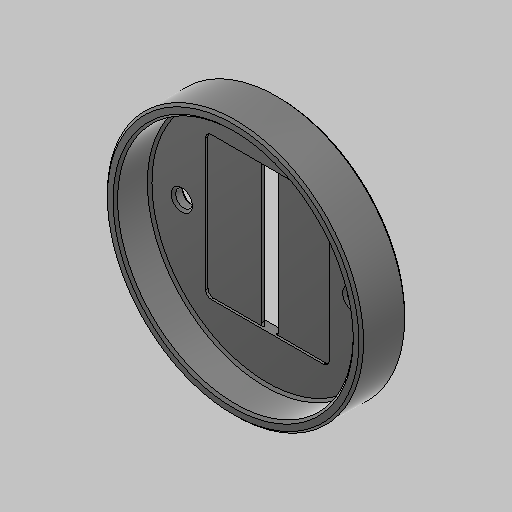
# Autodesk Inventor part: takumar-slit
Saved by Autodesk Inventor 2026 (Build 300175050, 175E)
## iProperties
Created: 2025-11-07
Part Number: takumar-slit
Material: ABS Plastic
Document SubType Name: Modeling
Designer: queezz
Density: 1.06 g/cm^3
Appearance: Smooth - Black
Author: queezz
Autodesk Inventor part; units mm, degrees
ref_plane "YZ Plane" through (0, 0, 0) normal (1, 0, 0) x (0, 1, 0)
ref_plane "XZ Plane" through (0, 0, 0) normal (0, 1, 0) x (-1, 0, 0)
ref_plane "XY Plane" through (0, 0, 0) normal (0, 0, 1) x (1, 0, 0)
sketch "Sketch1" plane through (0, 0, 0) normal (0, 0, 1) x (1, 0, 0)
  circle A0 centre (0, 0) radius 20.6
  circle A1 centre (0, 0) radius 22.4
  dimension "d0" = 41.2
  dimension "d1" = 1.8
  constraints: 2 centre point, 2 coincident
  measures "d0" diameter of A0
  measures "d1" radial gap between concentric circles of A0 A1
extrude "Extrusion1" add sketch "Sketch1" along normal blind 2 contours A0 | A1
extrude "Extrusion2" add sketch "Sketch1" along normal blind 8
sketch "Sketch2" plane through (0, 0, 2) normal (0, 0, 1) x (1, 0, 0)
  line L0 (-1.5, 12.5) -> (1.5, 12.5)
  line L1 (1.5, 12.5) -> (1.5, -12.5)
  line L2 (1.5, -12.5) -> (-1.5, -12.5)
  line L3 (-1.5, -12.5) -> (-1.5, 12.5)
  point P0 (0, 0)
  point P1 (0, 12.5)
  point P2 (1.5, 0)
  dimension "d6" = 3
  dimension "d7" = 25
  constraints: 8 end point, 2 midpoint, 2 parallel, 1 horizontal, 1 horizontal alignment, 1 perpendicular, 1 vertical alignment
  measures "d6" distance of L0.start L0.end
  measures "d7" distance of L0.end L1.end
extrude "Extrusion3" cut sketch "Sketch2" against normal through all
sketch "Sketch3" plane through (0, 0, 2) normal (0, 0, 1) x (1, 0, 0)
  line L0 (1.5, 12.5) -> (1.5, -12.5) projected
  line L1 (1.5, 12.5) -> (10.8, 12.5)
  line L2 (10.8, 12.5) -> (10.8, -12.5)
  line L3 (10.8, -12.5) -> (1.5, -12.5)
  line L4 (1.5, -12.5) -> (1.5, 12.5)
  point P0 (0, 0)
  dimension "d10" = 9.3
  constraints: 8 end point, 2 parallel, 1 horizontal, 1 perpendicular
  measures "d10" distance of L0.start L1.end
extrude "Extrusion4" cut sketch "Sketch3" against normal blind 0.4
mirror "Mirror1" about plane through (0, 0, 0) normal (1, 0, 0) of "Extrusion4"
chamfer "Chamfer1" distance 1 angle 45 2 edges at (1.5, 0, 0) (-1.5, 0, 0)
fillet "Fillet1" radius 0.4 4 edges at (-1.5, -12.5, 1.3) (1.5, -12.5, 1.3) (-1.5, 12.5, 1.3) (1.5, 12.5, 1.3)
fillet "Fillet2" radius 1 4 edges at (-10.8, 12.5, 1.8) (10.8, 12.5, 1.8) (10.8, -12.5, 1.8) (-10.8, -12.5, 1.8)
chamfer "Chamfer2" distance 0.4 angle 45 6 edges at (-22.4, 0, 8) (-20.6, 0, 8) (-20.6, 0, 2) (-22.4, 0, 0) (0, 12.5, 0) (0, -12.5, 0)
sketch "Sketch4" plane through (0, 0, 0) normal (0, 0, -1) x (-1, 0, 0)
  line L0 (15, 0) -> (-15, 0) construction
  point P0 (0, 0)
  point P1 (0, 0)
  dimension "d21" = 30
  constraints: 3 coincident, 2 end point, 1 horizontal, 1 midpoint
  measures "d21" distance of L0.start L0.end
hole "Hole1" at (-15, 0, 0) at (15, 0, 0) direction (0, 0, 1) diameter 2.9 end through all
chamfer "Chamfer3" distance 0.4 angle 45 4 edges at (15, -1.45, 0) (-15, -1.45, 0) (15, -1.45, 2) (-15, -1.45, 2)
body "Solid1"
